Handle (Autodesk Fusion 360 design; units mm, degrees)
Autodesk Fusion 360 part; units mm, degrees
sketch "草图1" plane through (0, 0, 0) normal (0, 0, 1) x (1, 0, 0)
  circle A0 centre (0, 0) radius 10
  circle A1 centre (0, 0) radius 3.275
  dimension "d1" = 20
  dimension "d2" = 6.55
  constraint coincident A0.centre A1.centre
  measures "d1" diameter of A0
  measures "d2" diameter of A1
extrude "拉伸1" add sketch "草图1" along normal blind 20
sketch "草图2" plane through (0, 0, 20) normal (0, 0, 1) x (-1, 0, 0)
  circle A0 centre (0, 0) radius 3.275
  circle A1 centre (0, 0) radius 10
  circle A2 centre (0, 0) radius 6
  dimension "d5" = 12
  constraint concentric A0 A2
  measures "d5" diameter of A2
extrude "拉伸2" add sketch "草图2" along normal blind 50 contours A1
extrude "Extrude3" add 1 faces at (-5.0571, 0.4608, 20) along direction (0, 0, 1) blind 5
sketch "Sketch3" plane through (0, 0, 70) normal (0, 0, 1) x (-1, 0, 0)
  circle A0 centre (0, 0) radius 6
  circle A1 centre (0, 0) radius 10
  circle A2 centre (0, 0) radius 15
  dimension "d11" = 30
  constraint coincident A0.centre A1.centre
  measures "d11" diameter of A2
extrude "Extrude4" add sketch "Sketch3" against normal blind 70 contours A2
chamfer "Chamfer2" distance 5 angle 75 1 edges at (13.9849, -5.4242, 0) measured on face at (-11.0236, 0.9079, 0)
extrude "Extrude5" add 1 faces at (-11.9442, 0.7452, 70) along direction (0, 0, 1) blind 5
chamfer "Chamfer3" distance 0.5 angle 45 2 edges at (-3.0534, 1.1843, 25) (-3.0534, 1.1843, 0) 1 faces at (-11.9442, 0.7452, 75) measured on face at (-5.0571, 0.4608, 25) measured on face at (3.2709, -0.1632, 16.6667)
chamfer "Chamfer1" [suppressed]
